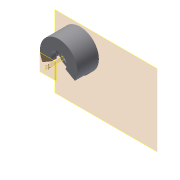
# Autodesk Inventor part: 101_Huawei_FilterLens_Adapter_Thread
Saved by Autodesk Inventor 2019 (Build 230136000, 136)
## iProperties
Created: 2019-06-17
Part Number: 101_Huawei_FilterLens_Adapter_Thread
Material: Generic
Document SubType Name: Modeling
Designer: diederichbenedict
Density: 1 g/cm^3
Appearance: Default
Author: diederichbenedict
Autodesk Inventor part; units mm, degrees
ref_plane "XZ Plane" through (0, 0, 0) normal (0, 1, 0) x (-1, 0, 0)
ref_plane "XY Plane" through (0, 0, 0) normal (0, 0, 1) x (1, 0, 0)
ref_plane "Work Plane1" through (0, 0, 0) normal (0, 0, 1) x (1, 0, 0)
ref_plane "Work Plane2" through (0, -6, 25.4) normal (0, 0, 1) x (1, 0, 0)
sketch "Sketch1" plane through (0, -6, 25.4) normal (0, 0, 1) x (1, 0, 0)
  point P0 (0, 6)
  point P1 (0, 6)
  constraints: 1 coincident
ref_plane "Work Plane3" through (0, 0, 25.4) normal (1, 0, 0) x (0, 1, 0)
sketch "Sketch2" plane through (0, 0, 25.4) normal (1, 0, 0) x (0, 1, 0)
  line L0 (12.6, -22.1) -> (12.6, -27.1) construction
  line L1 (8.75, -15.4) -> (8.75, -20.1) construction
  line L2 (-8.75, -15.4) -> (8.75, -15.4) construction
  arc A0 (-8.75, -20.1) -> (8.75, -20.1) centre (0, 0) ccw construction
  line L3 (-6, 0) -> (6, 0) construction
  line L4 (12.8, -25.4) -> (12.8, -21.9)
  line L5 (9.75, -20.7) -> (9.75, -15.0193)
  line L6 (9.75, -15.0193) -> (9.75, -12.4)
  line L7 (9.75, -12.4) -> (6.2, -12.4)
  line L8 (6.2, -12.4) -> (6.2, -8.4)
  line L9 (6.2, -8.4) -> (14.8, -8.4)
  line L10 (14.8, -8.4) -> (14.8, -25.4)
  line L11 (14.8, -25.4) -> (12.8, -25.4)
  line L12 (6, 0) -> (6, -15.4)
  line L13 (0, 0) -> (0, -25.4)
  line L14 (12.8, -21.9) -> (12.8, -20.7)
  line L15 (12.8, -20.7) -> (9.75, -20.7)
  line L16 (13.9634, -25.4) -> (8.8415, -25.4) projected
  dimension "d0" = 1
  dimension "d1" = 0.2
  dimension "d3" = 2
  dimension "d6" = 3
  dimension "d7" = 0.2
  dimension "d8" = 4
  dimension "d12" = 4.7
  constraints: 28 end point, 6 perpendicular, 6 vertical, 2 point on circle, 2 point on line, 1 centre point, 8 other
  measures "d0" distance between parallel lines of L1 L5
  measures "d1" distance between parallel lines of L0 L4
  measures "d3" distance between parallel lines of L4 L10
  measures "d6" distance between parallel lines of L2 L7
  measures "d7" distance between parallel lines of L12 L8
  measures "d8" distance between parallel lines of L7 L9
  measures "d12" distance between parallel lines of L15 L11
revolve "Revolution1" add sketch "Sketch2" angle 240 mid plane about axis through (0, 0, 25.4) along (0, -0.0000003, -1)
sketch "Sketch3" plane through (-12.8172, -7.4, 0) normal (0.5, -0.8660254, 0.0000002) x (0.8660254, 0.5, -0.0000004)
  line L0 (2, 0) -> (2, 4.7) projected
  line L1 (5.05, 4.7) -> (5.05, 13) projected
  line L2 (5.05, 13) -> (8.6, 13) projected
  line L3 (8.6, 13) -> (8.6, 17) projected
  line L4 (8.6, 17) -> (0, 17) projected
  line L5 (0, 17) -> (0, 0) projected
  line L6 (0, 0) -> (2, 0) projected
  line L7 (5.05, 4.7) -> (5.05, 13) projected
  line L8 (5.05, 4.7) -> (0, 4.7)
  line L9 (14.8, -5.08) -> (14.8, 30.48) projected
  line L10 (2, 4.7) -> (5.05, 4.7) projected
  line L11 (2, 0) -> (2, 4.7) projected
  line L12 (0, 4.7) -> (2, 4.7)
  line L13 (2, 4.7) -> (2, 0)
  line L14 (2, 0) -> (0, 0)
  line L15 (0, 0) -> (0, 4.7)
  point P0 (14.8, 0)
  constraints: 10 end point, 2 parallel, 2 perpendicular, 1 horizontal, 1 point on line
revolve "Revolution2" add sketch "Sketch3" angle 360 about axis through (0, 0, -10) along (-0.0000001, 0.0000002, 1) contours L6 L5 L8 L0
body "Solid1"
